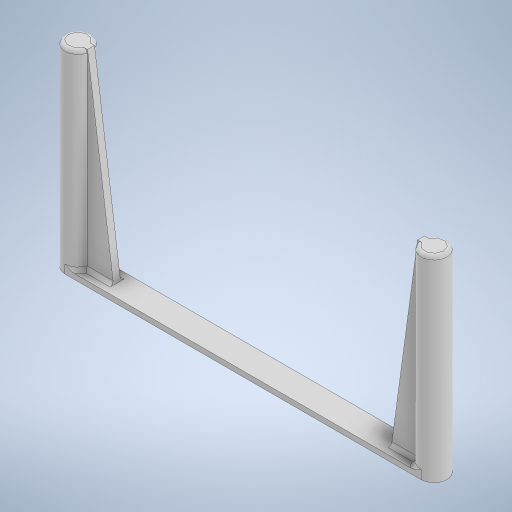
# Autodesk Inventor part: Soporte Platos
Saved by Autodesk Inventor 2024 (Build 280153000, 153)
## iProperties
Created: 2025-02-22
Part Number: Soporte Platos
Material: Genérico
Document SubType Name: Modeling
Designer: sergi
Density: 1 g/cm^3
Appearance: Valor por defecto
Author: sergi
Autodesk Inventor part; units mm, degrees
ref_plane "YZ Plane" through (0, 0, 0) normal (1, 0, 0) x (0, 1, 0)
ref_plane "XZ Plane" through (0, 0, 0) normal (0, 1, 0) x (-1, 0, 0)
ref_plane "XY Plane" through (0, 0, 0) normal (0, 0, 1) x (1, 0, 0)
sketch "Boceto1" plane through (0, 0, 0) normal (0, 1, 0) x (-1, 0, 0)
  line L0 (0, 0) -> (220, 0)
  line L1 (220, 0) -> (220, -760)
  line L2 (220, -760) -> (0, -760)
  line L3 (0, -760) -> (0, 0)
  dimension "d0" = 760
  dimension "d1" = 220
  constraints: 8 end point, 2 parallel, 1 horizontal, 1 perpendicular
  measures "d0" distance of L0.end L1.end
  measures "d1" distance of L1.end L2.end
extrude "Extrusión1" add sketch "Boceto1" along normal blind 3
sketch "Boceto3" plane through (0, 3, 0) normal (0, 1, 0) x (1, 0, 0)
  line L0 (0, 760) -> (-220, 760) projected
  line L1 (-220, 760) -> (-220, 0) projected
  line L2 (-220, 0) -> (0, 0) projected
  line L3 (0, 0) -> (0, 760) projected
  line L4 (-20, 20) -> (-200, 20)
  line L5 (-200, 20) -> (-200, 740)
  line L6 (-200, 740) -> (-20, 740)
  line L7 (-20, 740) -> (-20, 20)
  line L8 (0, 20) -> (-220, 20)
  line L9 (-220, 20) -> (-220, 35)
  line L10 (-220, 35) -> (0, 35)
  line L11 (0, 35) -> (0, 20)
  dimension "d4" = 20
  dimension "d5" = 15
  constraints: 16 end point, 3 point on line, 2 parallel, 1 horizontal, 1 perpendicular, 3 other
  measures "d4" distance between parallel lines of L2 L4
  measures "d5" distance of L8.end L9.end
extrude "Extrusión2" add sketch "Boceto3" along normal blind 3 contours L3 L8 L7 L10 | L10 L5 L8 L1 | L7 L4 L5 L10
sketch "Boceto4" plane through (0, 6, 0) normal (0, 1, 0) x (1, 0, 0)
  line L0 (-220, 35) -> (-220, 20) projected
  line L1 (-220, 20) -> (0, 20) projected
  line L2 (0, 20) -> (0, 35) projected
  line L3 (0, 35) -> (-220, 35) projected
  circle A0 centre (-7.5, 27.5) radius 7.5
  line L4 (0, 35) -> (-220, 35) projected
  line L5 (0, 20) -> (0, 35) projected
  circle A1 centre (-212.5, 27.5) radius 7.5
  line L6 (-220, 35) -> (-220, 20) projected
  point P0 (0, 0)
  dimension "d8" = 15
  dimension "d9" = 15
  constraints: 4 tangent, 2 centre point
  measures "d8" diameter of A0
  measures "d9" diameter of A1
extrude "Extrusión3" add sketch "Boceto4" along normal blind 110 contours A1 | A0
sketch "Boceto5" plane through (0, 6, 0) normal (0, 1, 0) x (1, 0, 0)
  circle A0 centre (-212.5, 27.5) radius 7.5 projected
  arc A1 (-7.5, 35) -> (-7.5, 20) centre (-7.5, 27.5) ccw projected
  line L0 (-7.5, 35) -> (-212.5, 35) projected
  arc A2 (-212.5, 20) -> (-212.5, 35) centre (-212.5, 27.5) ccw projected
  line L1 (-212.5, 20) -> (-7.5, 20) projected
  arc A3 (-212.5, 20) -> (-212.5, 35) centre (-212.5, 27.5) ccw projected
  line L2 (-205, 27.5) -> (-190, 27.5)
  line L3 (-190, 27.5) -> (-190, 29.5)
  line L4 (-190, 29.5) -> (-190, 25.5)
  line L5 (-190, 25.5) -> (-205.2716, 25.5)
  line L6 (-190, 29.5) -> (-205.2716, 29.5)
  arc A4 (-7.5, 20) -> (0, 27.5) centre (-7.5, 27.5) ccw projected
  line L7 (0, 20) -> (0, 27.5) projected
  line L8 (-7.5, 20) -> (0, 20) projected
  arc A5 (-220, 27.5) -> (-212.5, 20) centre (-212.5, 27.5) ccw projected
  line L9 (-220, 27.5) -> (-220, 20) projected
  line L10 (-220, 20) -> (-212.5, 20) projected
  point P0 (0, 0)
  dimension "d12" = 15
  dimension "d13" = 2
  dimension "d14" = 4
  constraints: 10 end point, 4 point on circle, 3 horizontal, 1 perpendicular, 1 point on line
  measures "d12" distance of L2.start L2.end
  measures "d13" distance of L2.end L3.end
  measures "d14" distance of L3.end L4.end
extrude "Extrusión4" add sketch "Boceto5" along normal up to surface (110 mm away) contours L2 L4 L5 A0 | A0 L6 L3 L2
chamfer "Chaflán2" distance 110 distance2 15 1 edges at (-190, 116, -27.5) measured on face at (-190, 115.5, -27.5)
ref_plane "Plano de trabajo1" through (-110, 0, 0) normal (1, 0, 0) x (0, 0, -1)
mirror "Simetría1" about plane through (-110, 0, 0) normal (1, 0, 0) of "Extrusión4", "Chaflán2"
fillet "Empalme1" radius 2 2 edges at (0, 116, -27.5) (-220, 116, -27.5)
sketch "Boceto6" plane through (0, 0, 0) normal (0, -1, 0) x (1, 0, 0)
  line L0 (-205, -29.5) -> (-205, -25.5) projected
  line L1 (-15, -25.5) -> (-15, -29.5) projected
  arc A0 (-12.6235, -29.5) -> (-12.6235, -25.5) centre (-7.5, -27.5) ccw projected
  arc A1 (-207.3765, -25.5) -> (-207.3765, -29.5) centre (-212.5, -27.5) ccw projected
  line L2 (-12.6235, -29.5) -> (-15, -29.5) projected
  line L3 (-15, -25.5) -> (-12.6235, -25.5) projected
  line L4 (-205, -25.5) -> (-207.3765, -25.5) projected
  line L5 (-207.3765, -29.5) -> (-205, -29.5) projected
  point P0 (0, 0)
hole "Agujero1" at (-212.5, 0, -27.5) at (-7.5, 0, -27.5) direction (0, 1, 0) diameter 4 depth 20 tip angle 118
sketch "Boceto8" plane through (0, 6, 0) normal (0, 1, 0) x (1, 0, 0)
  line L0 (-14.7284, 25.5) -> (-30, 25.5) projected
  line L1 (-30, 25.5) -> (-30, 29.5) projected
  line L2 (-30, 29.5) -> (-14.7284, 29.5) projected
  arc A0 (-7.5, 35) -> (-14.7284, 29.5) centre (-7.5, 27.5) ccw projected
  line L3 (-7.5, 35) -> (-212.5, 35) projected
  arc A1 (-205.2716, 29.5) -> (-212.5, 35) centre (-212.5, 27.5) ccw projected
  line L4 (-205.2716, 29.5) -> (-190, 29.5) projected
  line L5 (-190, 29.5) -> (-190, 25.5) projected
  line L6 (-190, 25.5) -> (-205.2716, 25.5) projected
  arc A2 (-212.5, 20) -> (-205.2716, 25.5) centre (-212.5, 27.5) ccw projected
  line L7 (-212.5, 20) -> (-7.5, 20) projected
  arc A3 (-14.7284, 25.5) -> (-7.5, 20) centre (-7.5, 27.5) ccw projected
  line L8 (-220, 35) -> (0, 35) projected
  line L9 (0, 35) -> (0, 760) projected
  line L10 (0, 760) -> (-220, 760) projected
  line L11 (-220, 760) -> (-220, 35) projected
  line L12 (0, 20) -> (-220, 20) projected
  line L13 (-220, 20) -> (-220, 0) projected
  line L14 (-220, 0) -> (0, 0) projected
  line L15 (0, 0) -> (0, 20) projected
  line L16 (0, 20) -> (0, 27.5) projected
  arc A4 (-14.7284, 25.5) -> (-14.7284, 29.5) centre (-7.5, 27.5) ccw projected
  line L17 (-220, 35) -> (0, 35) projected
  arc A5 (0, 27.5) -> (-7.5, 35) centre (-7.5, 27.5) ccw projected
  line L18 (0, 27.5) -> (0, 35) projected
  line L19 (0, 35) -> (-7.5, 35) projected
  arc A6 (-220, 27.5) -> (-212.5, 20) centre (-212.5, 27.5) ccw projected
  line L20 (-220, 27.5) -> (-220, 20) projected
  line L21 (-220, 20) -> (-212.5, 20) projected
  arc A7 (-212.5, 35) -> (-220, 27.5) centre (-212.5, 27.5) ccw projected
  line L22 (-212.5, 35) -> (-220, 35) projected
  line L23 (-220, 35) -> (-220, 27.5) projected
  point P0 (-220, 27.5)
  point P1 (-220, 27.5)
  point P2 (-220, 27.5)
  point P3 (-220, 27.5)
  point P4 (-212.5, 20)
extrude "Extrusión6" cut sketch "Boceto8" against normal blind 3 contours A4 L16 L12 | L12 L20 A6 | A4 L8 L18 | L23 L8 A7
fillet "Empalme3" radius 2 12 edges at (-207.9585, 6, -21.5313) (-197.6358, 6, -25.5) (-190, 6, -25.5) (-197.6358, 6, -29.5) (-190, 6, -29.5) (-207.9585, 6, -33.4687) (-30, 6.0001, -25.5) (-22.3642, 6, -25.5) (-12.0415, 6, -21.5313) (-12.0415, 6, -33.4687) (-30, 6.0001, -29.5) (-22.3642, 6, -29.5)
ref_plane "Plano de trabajo3" through (0, 3, 0) normal (0, 1, 0) x (1, 0, 0)
split "Dividir2" plane through (0, 3, 0) removes the side toward (0, -1, 0)
